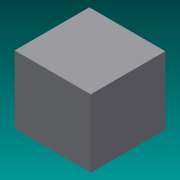
# Autodesk Inventor part: NL565050T-103J-PF
Saved by Autodesk Inventor 2015 (Build 190159000, 159)
## iProperties
Created: 2014-10-18
Part Number: NL565050T-103J-PF
Material: Generic
Document SubType Name: Modeling
Designer: Sawaiz Syed
Density: 1 g/cm^3
Appearance: Default
Author: Sawaiz Syed
Autodesk Inventor part; units mm, degrees
ref_plane "YZ Plane" through (0, 0, 0) normal (1, 0, 0) x (0, 1, 0)
ref_plane "XZ Plane" through (0, 0, 0) normal (0, 1, 0) x (-1, 0, 0)
ref_plane "XY Plane" through (0, 0, 0) normal (0, 0, 1) x (1, 0, 0)
sketch "Sketch1" plane through (0, 0, 0) normal (0, 0, 1) x (1, 0, 0)
  line L0 (-2.8, 2.75) -> (2.8, 2.75)
  line L1 (2.8, 2.75) -> (2.8, -2.75)
  line L2 (2.8, -2.75) -> (-2.8, -2.75)
  line L3 (-2.8, -2.75) -> (-2.8, 2.75)
  line L4 (-2.8, 2.75) -> (2.8, -2.75) construction
  line L5 (2.8, 2.75) -> (-2.8, -2.75) construction
  point P0 (0, 0)
  dimension "d0" = 5.6
  dimension "d1" = 5.5
  constraints: 12 end point, 2 midpoint, 2 parallel, 1 horizontal, 1 perpendicular
  measures "d0" distance of L1.end L2.end
  measures "d1" distance of L0.end L1.end
extrude "Extrusion1" add sketch "Sketch1" along normal blind 5
body "Solid1"
